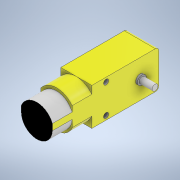
# Autodesk Inventor part: motorDC
Saved by Autodesk Inventor 2020 (Build 240168000, 168)
## iProperties
Created: 2020-04-18
Part Number: motorDC
Material: Genérico
Document SubType Name: Modeling
Designer: eduardoADM
Density: 1 g/cm^3
Appearance: Padrão
Author: eduardoADM
Autodesk Inventor part; units mm, degrees
ref_plane "YZ Plane" through (0, 0, 0) normal (1, 0, 0) x (0, 1, 0)
ref_plane "XZ Plane" through (0, 0, 0) normal (0, 1, 0) x (-1, 0, 0)
sketch "Esboço1" plane through (0, 0, 0) normal (0, 0, 1) x (1, 0, 0)
  line L0 (0, 0) -> (18.8, 0)
  line L1 (18.8, 0) -> (18.8, 22.5)
  line L2 (18.8, 22.5) -> (0, 22.5)
  line L3 (0, 22.5) -> (0, 0)
  dimension "d0" = 18.8
  dimension "d1" = 22.5
  constraints: 8 end point, 2 parallel, 1 horizontal, 1 perpendicular
  measures "d0" distance of L2.end L1.end
  measures "d1" distance of L1.end L0.end
extrude "Extrusão1" add sketch "Esboço1" along normal blind 64.2
sketch "Esboço2" plane through (18.8, 0, 0) normal (1, 0, 0) x (0, 0, -1)
  line L0 (0, 0) -> (-64.2, 0) projected
  line L1 (0, 0) -> (0, 11.25)
  line L2 (0, 0) -> (0, 22.5) projected
  line L3 (0, 11.25) -> (-11.2, 11.25)
  circle A0 centre (-11.2, 11.25) radius 2.7
  dimension "d4" = 11.25
  dimension "d5" = 11.2
  dimension "d6" = 5.4
  constraints: 4 end point, 1 centre point, 1 coincident, 1 midpoint, 1 perpendicular
  measures "d4" distance of L0.start L1.end
  measures "d5" distance of L1.end L3.end
  measures "d6" diameter of A0
extrude "Extrusão2" add sketch "Esboço2" along normal blind 1.1
sketch "Esboço3" plane through (19.9, 11.25, 11.2) normal (1, 0, 0) x (0, 0, -1)
  circle A0 centre (0, 0) radius 1.8
  point P0 (11.2, -11.25)
  dimension "d9" = 3.6
  constraints: 1 centre point
  measures "d9" diameter of A0
extrude "Extrusão3" add sketch "Esboço3" along normal blind 7.9
ref_plane "Plano de trabalho1" through (9.4, 0, 0) normal (1, 0, 0) x (0, 0, -1)
mirror "Espelhamento1" about plane through (9.4, 0, 0) normal (1, 0, 0) of "Extrusão3", "Extrusão2"
fillet "Arredondamento1" radius 2 1 edges at (9.4, 22.5, 0)
fillet "Arredondamento2" radius 2 1 edges at (9.4, 0, 0)
sketch "Esboço4" plane through (18.8, 0, 64.2) normal (1, 0, 0) x (0, 0, -1)
  line L0 (64.2, 0) -> (32.4, 0)
  line L1 (62.2, 0) -> (0, 0) projected
  line L2 (32.4, 0) -> (32.4, 2.5)
  circle A0 centre (32.4, 2.5) radius 1.5
  line L3 (32.4, 2.5) -> (32.4, 20)
  circle A1 centre (32.4, 20) radius 1.5
  dimension "d15" = 31.8
  dimension "d16" = 2.5
  dimension "d17" = 3
  dimension "d18" = 17.5
  dimension "d19" = 3
  constraints: 6 end point, 2 centre point, 2 coincident, 2 vertical, 1 point on line
  measures "d15" distance of L0.start L0.end
  measures "d16" distance of L0.end L2.end
  measures "d17" diameter of A0
  measures "d18" distance of L3.start L3.end
  measures "d19" diameter of A1
extrude "Extrusão4" cut sketch "Esboço4" against normal through all
sketch "Esboço5" plane through (0, 0, 64.2) normal (0, 0, 1) x (1, 0, 0)
  line L0 (18.8, 22.5) -> (0, 22.5)
  line L1 (0, 22.5) -> (18.8, 22.5)
  line L2 (18.8, 22.5) -> (18.8, 0)
  line L3 (18.8, 0) -> (0, 0)
  line L4 (0, 0) -> (0, 22.5)
  arc A0 (18.8, 17.831338) -> (0, 17.831338) centre (9.4, 10.702573) ccw
  point P0 (9.4, 22.5)
  constraints: 8 end point, 2 parallel, 2 point on circle, 2 point on line, 1 centre point, 1 horizontal, 1 perpendicular
extrude "Extrusão5" cut sketch "Esboço5" against normal blind 23.8 contours L2 A0 L0 | A0 L4 L0
sketch "Esboço6" plane through (0, 0, 64.2) normal (0, 0, 1) x (1, 0, 0)
  line L0 (0, 22.508504) -> (18.8, 22.508504)
  line L1 (18.8, 22.508504) -> (18.8, 0)
  line L2 (18.8, 0) -> (0, 0)
  line L3 (0, 0) -> (0, 22.508504)
  arc A0 (0, 6.267075) -> (18.8, 6.372369) centre (9.378542, 10.150894) ccw
  point P0 (9.357085, 0)
  point P1 (9.4, 0)
  constraints: 8 end point, 2 parallel, 2 point on circle, 2 point on line, 1 centre point, 1 horizontal, 1 perpendicular
extrude "Extrusão6" cut sketch "Esboço6" against normal blind 23.8 contours A0 L2 L3 | L1 L2 A0
sketch "Esboço7" plane through (0, 0, 64.2) normal (0, 0, 1) x (1, 0, 0)
  line L0 (0, 22.5) -> (9.4, 22.5)
  line L1 (0, 22.5) -> (18.8, 22.5)
  line L2 (18.8, 22.5) -> (18.8, 0)
  line L3 (18.8, 0) -> (0, 0)
  line L4 (0, 0) -> (0, 22.5)
  arc A0 (18.8, 14.455208) -> (0, 14.564328) centre (9.378542, 10.812909) ccw
  constraints: 8 end point, 2 parallel, 2 point on circle, 2 point on line, 1 centre point, 1 horizontal, 1 perpendicular
extrude "Extrusão7" cut sketch "Esboço7" against normal blind 11.9 contours L0 L1 L2 A0 L4
sketch "Esboço9" plane through (0, 0, 64.2) normal (0, 0, 1) x (1, 0, 0)
  line L0 (0, 20.5) -> (0, 2)
  line L1 (18.8, 13.95) -> (18.8, 8.55)
  arc A0 (0, 11.25) -> (18.8, 11.25) centre (9.4, 10.967634) ccw
  line L2 (0, 20.5) -> (0, 22.5)
  line L3 (0, 22.5) -> (18.8, 22.5)
  line L4 (18.8, 22.5) -> (18.8, 0)
  line L5 (18.8, 0) -> (0, 0)
  line L6 (0, 0) -> (0, 22.5)
  point P0 (18.8, 10.685268)
  point P1 (0, 10.685268)
  constraints: 8 end point, 2 midpoint, 2 parallel, 2 point on circle, 1 centre point, 1 horizontal, 1 perpendicular
sketch "Esboço9 outline for Extrusão8" plane through (0, 0, 64.2) normal (0, 0, 1) x (1, 0, 0)
  line L0 (0, 0) -> (18.8, 0)
  line L1 (0, 2) -> (0, 0)
  line L2 (0, 10.685268) -> (0, 2)
  arc A0 (18.8, 10.685268) -> (0, 10.685268) centre (9.4, 10.967634) cw
  line L3 (18.8, 8.55) -> (18.8, 10.685268)
  line L4 (18.8, 0) -> (18.8, 8.55)
extrude "Extrusão8" cut sketch "Esboço9 outline for Extrusão8" against normal blind 11.9
